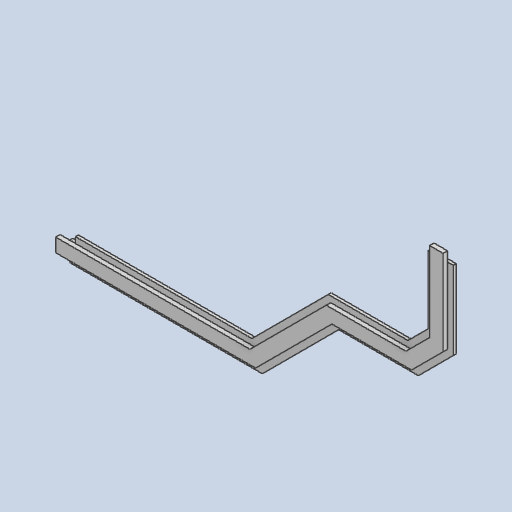
# Autodesk Inventor part: left_line
Saved by Autodesk Inventor 2022 (Build 260153000, 153)
## iProperties
Created: 2024-07-10
Part Number: left_line
Material: Типовые
Document SubType Name: Modeling
Designer: Капустяник Андрей
Density: 1 g/cm^3
Appearance: По умолчанию
Author: Капустяник Андрей
Autodesk Inventor part; units mm, degrees
ref_plane "YZ Plane" through (0, 0, 0) normal (1, 0, 0) x (0, 1, 0)
ref_plane "XZ Plane" through (0, 0, 0) normal (0, 1, 0) x (-1, 0, 0)
ref_plane "XY Plane" through (0, 0, 0) normal (0, 0, 1) x (1, 0, 0)
sketch "Эскиз1" plane through (0, 0, 0) normal (0, 0, 1) x (1, 0, 0)
  line L0 (-136.1512, -7) -> (-131.1512, -2) projected
  line L1 (-131.1512, -2) -> (-99.224, -2) projected
  line L2 (-19, -2) -> (-19, -22) projected
  line L3 (-19, -22) -> (-24, -27) projected
  line L4 (-24, -27) -> (-30.8711, -27) projected
  line L5 (-136.1512, -27) -> (-136.1512, -7) projected
  line L6 (-141.1512, -58) -> (-75.0711, -58) projected
  line L7 (-75.0711, -58) -> (-49.0711, -32) projected
  line L8 (-49.0711, -32) -> (-21.9289, -32) projected
  line L9 (-21.9289, -32) -> (-14, -24.0711) projected
  line L10 (-14, -24.0711) -> (-14, 3) projected
  line L11 (-133.2223, 3) -> (-14, 3) projected
  line L12 (-133.2223, 3) -> (-141.1512, -4.9289) projected
  line L13 (-141.1512, -58) -> (-141.1512, -4.9289) projected
  line L14 (-44.9289, -42) -> (-24.8579, -42) projected
  line L15 (-24.8579, -42) -> (-45.8579, -63) projected
  line L16 (-45.8579, -63) -> (-65.9289, -63) projected
  line L17 (-65.9289, -63) -> (-44.9289, -42) projected
  line L18 (-4, 3) -> (-9, 3) projected
  line L19 (-9, 3) -> (-9, -26.1421) projected
  line L20 (-9, -26.1421) -> (-19.8579, -37) projected
  line L21 (-19.8579, -37) -> (-47, -37) projected
  line L22 (-47, -37) -> (-73, -63) projected
  line L23 (-73, -63) -> (-141.1512, -63) projected
  line L24 (-141.1512, -67.9) -> (-141.1512, -63) projected
  line L25 (-47.0828, -36.8) -> (-19.9407, -36.8)
  line L26 (-19.9407, -36.8) -> (-9.2, -26.0593)
  line L27 (-9.2, -26.0593) -> (-9.2, 3.2)
  line L28 (-9.2, 3.2) -> (3.2, 3.2)
  line L29 (3.2, 3.2) -> (3.2, -31.1955)
  line L30 (3.2, -31.1955) -> (-40.7045, -75.1)
  line L31 (-40.7045, -75.1) -> (-141.3512, -75.1)
  line L32 (-141.3512, -75.1) -> (-141.3512, -62.8)
  line L33 (-141.3512, -62.8) -> (-73.0828, -62.8)
  line L34 (-73.0828, -62.8) -> (-47.0828, -36.8)
  line L35 (-21.8461, -32.2) -> (-48.9882, -32.2)
  line L36 (-48.9882, -32.2) -> (-74.9882, -58.2)
  line L37 (-74.9882, -58.2) -> (-141.3512, -58.2)
  line L38 (-141.3512, -58.2) -> (-141.3512, -4.8461)
  line L39 (-141.3512, -4.8461) -> (-133.3051, 3.2)
  line L40 (-133.3051, 3.2) -> (-13.8, 3.2)
  line L41 (-13.8, 3.2) -> (-13.8, -24.1539)
  line L42 (-13.8, -24.1539) -> (-21.8461, -32.2)
  line L43 (-9, 3) -> (-14, 3)
  line L44 (-141.1512, -63) -> (-141.1512, -58)
  line L45 (-99.224, -2) -> (-93.5671, -2) projected
  line L46 (-93.5671, -2) -> (-86.696, -2) projected
  line L47 (-86.696, -2) -> (-81.0391, -2) projected
  line L48 (-81.0391, -2) -> (-74.168, -2) projected
  line L49 (-74.168, -2) -> (-68.5111, -2) projected
  line L50 (-68.5111, -2) -> (-61.64, -2) projected
  line L51 (-61.64, -2) -> (-55.9831, -2) projected
  line L52 (-55.9831, -2) -> (-49.112, -2) projected
  line L53 (-49.112, -2) -> (-43.4551, -2) projected
  line L54 (-43.4551, -2) -> (-36.584, -2) projected
  line L55 (-36.584, -2) -> (-30.9271, -2) projected
  line L56 (-30.9271, -2) -> (-19, -2) projected
  line L57 (-30.8711, -27) -> (-36.528, -27) projected
  line L58 (-36.528, -27) -> (-43.3991, -27) projected
  line L59 (-43.3991, -27) -> (-49.056, -27) projected
  line L60 (-49.056, -27) -> (-55.9271, -27) projected
  line L61 (-55.9271, -27) -> (-61.584, -27) projected
  line L62 (-61.584, -27) -> (-68.4551, -27) projected
  line L63 (-68.4551, -27) -> (-74.112, -27) projected
  line L64 (-74.112, -27) -> (-80.9831, -27) projected
  line L65 (-80.9831, -27) -> (-86.64, -27) projected
  line L66 (-86.64, -27) -> (-93.5111, -27) projected
  line L67 (-93.5111, -27) -> (-99.168, -27) projected
  line L68 (-99.168, -27) -> (-106.0391, -27) projected
  line L69 (-106.0391, -27) -> (-111.696, -27) projected
  line L70 (-111.696, -27) -> (-136.1512, -27) projected
  line L71 (-43.6868, -67.9) -> (-141.1512, -67.9) projected
  line L72 (-4, -28.2132) -> (-43.6868, -67.9) projected
  line L73 (-4, 3) -> (-4, -28.2132) projected
  point P0 (-9.2, 3)
  point P1 (-13.8, 3)
  point P2 (-141.1512, -58.2)
  point P3 (-141.1512, -62.8)
  dimension "d15" = 0.2
  dimension "d16" = 0.2
  constraints: 40 end point, 1 horizontal, 1 perpendicular, 12 other
  measures "d15" distance between parallel lines of L21 L25
  measures "d16" distance between parallel lines of L8 L35
extrude "Выдавливание1" add sketch "Эскиз1" against normal blind 1.5 contours L37 L36 L35 L42 L41 L43 L27 L26 L25 L34 L33 L44
sketch "Эскиз2" plane through (0, 0, 0) normal (0, 0, 1) x (1, 0, 0)
  line L0 (-9.2, -26.0593) -> (-9.2, 3) projected
  line L1 (-9.2, 3) -> (-13.8, 3) projected
  line L2 (-13.8, 3) -> (-13.8, -24.1539) projected
  line L3 (-13.8, -24.1539) -> (-21.8461, -32.2) projected
  line L4 (-21.8461, -32.2) -> (-48.9882, -32.2) projected
  line L5 (-48.9882, -32.2) -> (-74.9882, -58.2) projected
  line L6 (-74.9882, -58.2) -> (-141.1512, -58.2) projected
  line L7 (-141.1512, -58.2) -> (-141.1512, -62.8) projected
  line L8 (-141.1512, -62.8) -> (-73.0828, -62.8) projected
  line L9 (-73.0828, -62.8) -> (-47.0828, -36.8) projected
  line L10 (-47.0828, -36.8) -> (-19.9407, -36.8) projected
  line L11 (-19.9407, -36.8) -> (-9.2, -26.0593) projected
  line L12 (-7.2, -26.8877) -> (-7.2, 5)
  line L13 (-7.2, 5) -> (-15.8, 5)
  line L14 (-15.8, 5) -> (-15.8, -23.3255)
  line L15 (-15.8, -23.3255) -> (-22.6745, -30.2)
  line L16 (-22.6745, -30.2) -> (-49.8167, -30.2)
  line L17 (-49.8167, -30.2) -> (-75.8167, -56.2)
  line L18 (-75.8167, -56.2) -> (-143.1512, -56.2)
  line L19 (-143.1512, -56.2) -> (-143.1512, -64.8)
  line L20 (-143.1512, -64.8) -> (-72.2544, -64.8)
  line L21 (-72.2544, -64.8) -> (-46.2544, -38.8)
  line L22 (-46.2544, -38.8) -> (-19.1123, -38.8)
  line L23 (-19.1123, -38.8) -> (-7.2, -26.8877)
  line L24 (-138.1512, -66.9) -> (-138.1512, -63) projected
  line L25 (-138.1512, -64.8) -> (-137.8512, -64.8)
  line L26 (-137.8512, -64.8) -> (-137.8512, -56.2)
  line L27 (-5.3, 0) -> (-14, 0) projected
  line L28 (-7.2, 0) -> (-7.2, -0.3)
  line L29 (-7.2, -0.3) -> (-15.8, -0.3)
  dimension "d17" = 2
  dimension "d18" = 0.3
  dimension "d19" = 0.3
  constraints: 32 end point, 8 point on line, 2 perpendicular, 11 other
  measures "d17" distance between parallel lines of L11 L23
  measures "d18" distance of L25.start L25.end
  measures "d19" distance of L28.start L28.end
extrude "Выдавливание2" add sketch "Эскиз2" along normal blind 1 contours L11 L10 L9 L8 L26 L6 L5 L4 L3 L2 L29 L0 | L0 L29 L12 L23 L22 L21 L20 L26 L8 L9 L10 L11 | L2 L3 L4 L5 L6 L26 L18 L17 L16 L15 L14 L29
mirror "Зеркальное отражение1" about plane through (-72.5256, -32.55, 1) normal (0, 0, 1) of "Выдавливание2", "Выдавливание1"
sketch "Эскиз3" plane through (0, 0, -1.5) normal (0, 0, -1) x (-1, 0, 0)
  line L0 (163, 30) -> (-28, 30)
  line L1 (-28, 30) -> (-28, -127)
  line L2 (-28, -127) -> (163, -127)
  line L3 (163, -127) -> (163, 30)
  point P0 (0, 0)
  constraints: 8 end point, 2 parallel, 1 horizontal, 1 perpendicular
extrude "Выдавливание3" cut sketch "Эскиз3" against normal blind 2.5
sketch "Эскиз4" plane through (0, 0, 1) normal (0, 0, -1) x (-1, 0, 0)
  line L0 (39.0089, -22.15) -> (21.8668, -22.15) projected
  line L1 (21.8668, -22.15) -> (13.85, -14.1332) projected
  line L2 (13.85, -14.1332) -> (13.85, 3) projected
  line L3 (13.85, 3) -> (9.15, 3) projected
  line L4 (9.15, 3) -> (9.15, -16.08) projected
  line L5 (9.15, -16.08) -> (19.92, -26.85) projected
  line L6 (19.92, -26.85) -> (37.0621, -26.85) projected
  line L7 (37.0621, -26.85) -> (73.0621, -62.85) projected
  line L8 (73.0621, -62.85) -> (141.1512, -62.85) projected
  line L9 (141.1512, -62.85) -> (141.1512, -58.15) projected
  line L10 (141.1512, -58.15) -> (75.0089, -58.15) projected
  line L11 (75.0089, -58.15) -> (39.0089, -22.15) projected
  line L12 (9.15, -16.08) -> (9.15, -0.2) projected
  line L13 (6, -0.2) -> (9.15, -0.2) projected
  line L14 (6, -17.3848) -> (6, -0.2) projected
  line L15 (18.6152, -30) -> (6, -17.3848) projected
  line L16 (35.7574, -30) -> (18.6152, -30) projected
  line L17 (71.7574, -66) -> (35.7574, -30) projected
  line L18 (137.9512, -66) -> (71.7574, -66) projected
  line L19 (137.9512, -62.85) -> (137.9512, -66) projected
  line L20 (137.9512, -62.85) -> (73.0621, -62.85) projected
  line L21 (73.0621, -62.85) -> (37.0621, -26.85) projected
  line L22 (37.0621, -26.85) -> (19.92, -26.85) projected
  line L23 (19.92, -26.85) -> (9.15, -16.08) projected
  line L24 (13.85, -0.2) -> (13.85, -14.1332) projected
  line L25 (13.85, -14.1332) -> (21.8668, -22.15) projected
  line L26 (21.8668, -22.15) -> (39.0089, -22.15) projected
  line L27 (39.0089, -22.15) -> (75.0089, -58.15) projected
  line L28 (75.0089, -58.15) -> (137.9512, -58.15) projected
  line L29 (137.9512, -55) -> (137.9512, -58.15) projected
  line L30 (76.3137, -55) -> (137.9512, -55) projected
  line L31 (40.3137, -19) -> (76.3137, -55) projected
  line L32 (23.1716, -19) -> (40.3137, -19) projected
  line L33 (17, -12.8284) -> (23.1716, -19) projected
  line L34 (17, -0.2) -> (17, -12.8284) projected
  line L35 (13.85, -0.2) -> (17, -0.2) projected
  line L36 (137.9512, -58.15) -> (135.9512, -58.15)
  line L37 (135.9512, -58.15) -> (135.9512, -55)
  line L38 (135.9512, -55) -> (137.9512, -55)
  line L39 (137.9512, -55) -> (137.9512, -58.15)
  point P0 (0, 0)
  point P1 (135.9512, -58.15)
  dimension "d12" = 2
  constraints: 8 end point, 2 parallel, 1 horizontal, 1 perpendicular, 1 point on line
  measures "d12" distance of L37.end L38.end
extrude "Выдавливание4" cut sketch "Эскиз4" against normal blind 1 contours L37 L30 L29 L10
